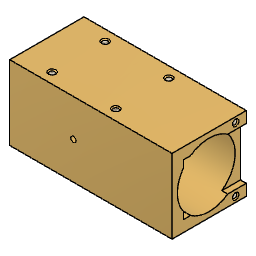
Anton_Buguev_MAM2021.01.01.000 (Autodesk Fusion 360 archive; units mm, degrees)
design "MAM2021.01.01.001"
Autodesk Fusion 360 part; units mm, degrees
sketch "Sketch1" plane through (0, 0, 0) normal (0, 1, 0) x (1, 0, 0)
  line L0 (38.25, 17.5) -> (-38.25, 17.5)
  line L1 (-38.25, 17.5) -> (-38.25, -17.5)
  line L2 (-38.25, -17.5) -> (38.25, -17.5)
  line L3 (38.25, -17.5) -> (38.25, 17.5)
  line L4 (38.25, 17.5) -> (-38.25, -17.5) construction
  line L5 (-38.25, 17.5) -> (38.25, -17.5) construction
  dimension "d1" = 76.5
  dimension "d2" = 35
  constraint horizontal L0
  constraint perpendicular L0 L1
  constraint parallel L0 L2
  constraint parallel L1 L3
  constraint coincident L4 origin
  constraint coincident L5 origin
  measures "d1" distance of L1.end L2.end
  measures "d2" distance of L0.end L1.end
extrude "Extrude1" add sketch "Sketch1" along normal blind 35
sketch "Sketch2" plane through (38.25, 0, 0) normal (1, 0, 0) x (0, 0, -1)
  line L0 (-17.5, 0) -> (17.5, 0)
  line L1 (17.5, 0) -> (17.5, 35)
  line L2 (17.5, 35) -> (-17.5, 35)
  line L3 (-17.5, 35) -> (-17.5, 0)
  circle A0 centre (0, 17.5) radius 15
  line L4 (0, 17.5) -> (17.5, 17.5) construction
  line L5 (17.5, 17.5) -> (17.5, 29.7)
  line L6 (17.5, 29.7) -> (-12, 29.7)
  line L7 (-12, 29.7) -> (-12, 5.3)
  line L8 (-12, 5.3) -> (17.5, 5.3)
  line L9 (17.5, 5.3) -> (17.5, 17.5)
  circle A1 centre (12.5, 32.5) radius 1.25 construction
  circle A2 centre (12.5, 2.5) radius 1.25 construction
  dimension "d5" = 30
  dimension "d6" = 17.5
  dimension "d7" = 17.5
  dimension "d8" = 12.2
  dimension "d9" = 29.5
  dimension "d10" = 24.4
  dimension "d11" = 2.5
  dimension "d12" = 2.5
  dimension "d13" = 5
  dimension "d14" = 2.5
  dimension "d15" = 5
  dimension "d16" = 2.5
  constraint coincident A0.centre L4.start
  constraint midpoint L1 L4.end
  constraint perpendicular L4 L5
  constraint perpendicular L5 L6
  constraint perpendicular L0 L7
  constraint coincident L1 L8.end
  constraint perpendicular L1 L8
  measures "d5" diameter of A0
  measures "d6" distance of L3 A0.centre
  measures "d7" distance of L0 A0.centre
  measures "d8" distance of L4.end L5.end
  measures "d9" distance of L5.end L6.end
  measures "d10" distance of L6.end L7.end
  measures "d11" diameter of A1
  measures "d12" distance of L2 A1.centre
  measures "d13" distance of L1 A1.centre
  measures "d14" diameter of A2
  measures "d15" distance of L1 A2.centre
  measures "d16" distance of L0 A2.centre
extrude "Extrude2" cut sketch "Sketch2" against normal blind 25.5 contours A0 L6 L7 L8 | A0 L8 | A0 L6 | A0 L7
extrude "Extrude3" cut sketch "Sketch2" against normal blind 2.75 contours L1 A0 L5 L6 L8 L9 | A0 L7 L8 | A0 L6 L7
sketch "Sketch3" plane through (-38.25, 0, 0) normal (-1, 0, 0) x (0, 0, 1)
  line L0 (-17.5, 0) -> (17.5, 0)
  line L1 (17.5, 0) -> (17.5, 35)
  line L2 (17.5, 35) -> (-17.5, 35)
  line L3 (-17.5, 35) -> (-17.5, 0)
  circle A0 centre (0, 17.5) radius 15
  line L4 (13.4987, 4.0013) -> (13.4987, 30.9987) construction
  line L5 (13.4987, 30.9987) -> (-13.4987, 30.9987) construction
  line L6 (-13.4987, 30.9987) -> (-13.4987, 4.0013) construction
  line L7 (-13.4987, 4.0013) -> (13.4987, 4.0013) construction
  circle A1 centre (-13.4987, 30.9987) radius 1.5
  circle A2 centre (13.4987, 30.9987) radius 1.5
  circle A3 centre (13.4987, 4.0013) radius 1.5
  circle A4 centre (-13.4987, 4.0013) radius 1.5
  point P0 (0, 17.5)
  dimension "d21" = 30
  dimension "d22" = 17.5
  dimension "d23" = 17.5
  dimension "d24" = 19.09
  dimension "d25" = 3
  dimension "d26" = 3
  dimension "d27" = 3
  dimension "d28" = 3
  constraint coincident P0 A0.centre
  constraint horizontal L5
  constraint coincident L5.end L6.start
  constraint coincident L4.end L5.start
  constraint coincident L4.start L7.end
  constraint coincident L6.end L7.start
  measures "d21" diameter of A0
  measures "d22" distance of L2 P0
  measures "d23" distance of L1 P0
  measures "d24" distance of L4.start P0
  measures "d25" diameter of A1
  measures "d26" diameter of A2
  measures "d27" diameter of A3
  measures "d28" diameter of A4
extrude "Extrude4" cut sketch "Sketch3" against normal blind 10 contours A0
sketch "Sketch4" plane through (-28.25, 0, 0) normal (-1, 0, 0) x (0, 0, 1)
  circle A0 centre (0, 17.5) radius 15
  circle A1 centre (0, 17.5) radius 12.5
  dimension "d31" = 25
  constraint concentric A0 A1
  measures "d31" diameter of A1
extrude "Extrude5" cut sketch "Sketch4" against normal blind 41 contours A1
sketch "Sketch5" plane through (0, 0, 17.5) normal (0, 0, 1) x (1, 0, 0)
  line L0 (-38.25, 0) -> (38.25, 0)
  line L1 (38.25, 0) -> (38.25, 35)
  line L2 (38.25, 35) -> (-38.25, 35)
  line L3 (-38.25, 35) -> (-38.25, 0)
  line L4 (-38.25, 17.5) -> (-8.25, 17.5) construction
  line L5 (-8.25, 17.5) -> (11.75, 17.5) construction
  circle A0 centre (-8.25, 17.5) radius 1.25
  circle A1 centre (11.75, 17.5) radius 2.5
  dimension "d34" = 30
  dimension "d35" = 20
  dimension "d36" = 2.5
  dimension "d37" = 5
  constraint midpoint L3 L4.start
  constraint perpendicular L3 L4
  constraint perpendicular L3 L5
  constraint coincident L4.end L5.start
  constraint coincident L5.end A1.centre
  measures "d34" distance of L4.start L4.end
  measures "d35" distance of L4.end L5.end
  measures "d36" diameter of A0
  measures "d37" diameter of A1
extrude "Extrude6" cut sketch "Sketch5" against normal blind 35 contours A0
extrude "Extrude7" cut sketch "Sketch5" along normal blind -20 and the other way blind 35 contours A1
sketch "Sketch6" plane through (0, 35, 0) normal (0, 1, 0) x (-1, 0, 0)
  line L0 (-38.25, 17.5) -> (-38.25, -17.5)
  line L1 (-38.25, -17.5) -> (38.25, -17.5)
  line L2 (38.25, -17.5) -> (38.25, 17.5)
  line L3 (38.25, 17.5) -> (-38.25, 17.5)
  circle A0 centre (23.25, -12.5) radius 1.5
  circle A1 centre (-6.75, -12.5) radius 1.5
  circle A2 centre (23.25, 12.5) radius 1.5
  circle A3 centre (-6.75, 12.5) radius 1.5
  dimension "d44" = 3
  dimension "d45" = 15
  dimension "d46" = 5
  dimension "d49" = -30
  dimension "d50" = 25
  measures "d44" diameter of A0
  measures "d45" distance of L2 A0.centre
  measures "d46" distance of L1 A0.centre
sketch "Sketch7" plane through (0, 0, 0) normal (0, -1, 0) x (1, 0, 0)
  line L0 (38.25, -17.5) -> (38.25, 17.5)
  line L1 (38.25, 17.5) -> (-38.25, 17.5)
  line L2 (-38.25, 17.5) -> (-38.25, -17.5)
  line L3 (-38.25, -17.5) -> (38.25, -17.5)
  circle A0 centre (-23.25, 12.5) radius 1.5
  circle A1 centre (6.75, 12.5) radius 1.5
  circle A2 centre (-23.25, -12.5) radius 1.5
  circle A3 centre (6.75, -12.5) radius 1.5
  dimension "d51" = 3
  dimension "d52" = 5
  dimension "d53" = 15
  dimension "d56" = 30
  dimension "d57" = -25
  measures "d51" diameter of A0
  measures "d52" distance of L1 A0.centre
  measures "d53" distance of L2 A0.centre
hole "Hole1" at (-38.25, 30.9987, 13.4987) at (-38.25, 30.9987, -13.4987) at (-38.25, 4.0013, -13.4987) at (-38.25, 4.0013, 13.4987) direction (1, 0, 0) diameter 2.529 depth 7 tip angle 118 countersink diameter 3.5 countersink angle 90
thread "Thread1" "ISO Metric profile 3.0 M3x0.5 6H" thread offset 0 thread depth 5
hole "Hole2" at (-23.25, 35, 12.5) at (6.75, 35, 12.5) at (6.75, 35, -12.5) at (-23.25, 35, -12.5) direction (0, -1, 0) diameter 2.529 depth 7 tip angle 118 countersink diameter 3.5 countersink angle 90
thread "Thread2" "ISO Metric profile 3.0 M3x0.5 6H" thread offset 0 thread depth 5
hole "Hole3" at (-23.25, 0, 12.5) at (-23.25, 0, -12.5) at (6.75, 0, -12.5) at (6.75, 0, 12.5) direction (0, 1, 0) diameter 2.529 depth 7 tip angle 118 countersink diameter 3.5 countersink angle 90
thread "Thread3" "ISO Metric profile 3.0 M3x0.5 6H" thread offset 0 thread depth 5
hole "Hole4" at (38.25, 32.5, -12.5) at (38.25, 2.5, -12.5) direction (-1, 0, 0) diameter 2.076 depth 5 tip angle 118 countersink diameter 3.05 countersink angle 90
thread "Thread4" "ISO Metric profile 2.5 M2.5x0.45 6H" thread offset 0 thread depth 4
equation "d24 = ( 38.18 / 2 ) * 1 mm"

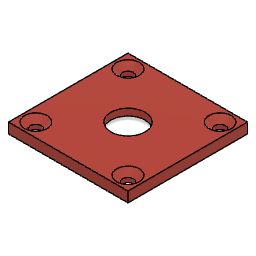
design "MAM2021.01.01.002"
Autodesk Fusion 360 part; units mm, degrees
sketch "Sketch1" plane through (0, 0, 0) normal (0, 1, 0) x (1, 0, 0)
  line L0 (17.5, -17.5) -> (-17.5, -17.5)
  line L1 (-17.5, -17.5) -> (-17.5, 17.5)
  line L2 (-17.5, 17.5) -> (17.5, 17.5)
  line L3 (17.5, 17.5) -> (17.5, -17.5)
  line L4 (17.5, -17.5) -> (-17.5, 17.5) construction
  line L5 (-17.5, -17.5) -> (17.5, 17.5) construction
  circle A0 centre (0, 0) radius 5
  dimension "d1" = 35
  dimension "d2" = 35
  dimension "d3" = 10
  constraint horizontal L0
  constraint perpendicular L0 L1
  constraint parallel L0 L2
  constraint parallel L1 L3
  constraint coincident L4 A0.centre
  constraint coincident L5 A0.centre
  constraint coincident A0.centre origin
  measures "d1" distance of L1.end L2.end
  measures "d2" distance of L0.end L1.end
  measures "d3" diameter of A0
extrude "Extrude1" add sketch "Sketch1" along normal blind 3
sketch "Sketch2" plane through (0, 3, 0) normal (0, 1, 0) x (-1, 0, 0)
  circle A0 centre (0, 0) radius 5
  line L0 (-17.5, -17.5) -> (17.5, -17.5)
  line L1 (17.5, -17.5) -> (17.5, 17.5)
  line L2 (17.5, 17.5) -> (-17.5, 17.5)
  line L3 (-17.5, 17.5) -> (-17.5, -17.5)
  line L4 (-13.4987, -13.4987) -> (13.4987, -13.4987) construction
  line L5 (13.4987, -13.4987) -> (13.4987, 13.4987) construction
  line L6 (13.4987, 13.4987) -> (-13.4987, 13.4987) construction
  line L7 (-13.4987, 13.4987) -> (-13.4987, -13.4987) construction
  circle A1 centre (0, 0) radius 10
  dimension "d6" = 19.09
  dimension "d7" = 20
  constraint coincident A0.centre A1.centre
  constraint horizontal L4
  constraint concentric A0 A1
  measures "d6" distance of L4.start A0.centre
  measures "d7" diameter of A1
hole "Hole1" at (13.4987, 3, -13.4987) at (-13.4987, 3, -13.4987) at (-13.4987, 3, 13.4987) at (13.4987, 3, 13.4987) direction (0, -1, 0) diameter 3.2 end through all countersink diameter 6.6 countersink angle 90
extrude "Extrude2" cut sketch "Sketch2" along normal blind -3 and the other way blind 2 contours A1
equation "d6 = ( 38.18 / 2 ) * 1 mm"

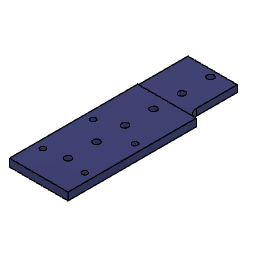
design "MAM2021.01.01.004"
Autodesk Fusion 360 part; units mm, degrees
sketch "Sketch1" plane through (0, 0, 0) normal (0, 1, 0) x (1, 0, 0)
  line L0 (0, 0) -> (17.5, 0) construction
  line L1 (17.5, -53.25) -> (17.5, 53.25)
  line L2 (17.5, 53.25) -> (-17.5, 53.25)
  line L3 (-17.5, 53.25) -> (-17.5, -23.25)
  line L4 (-17.5, -23.25) -> (-17.5, -28.75) construction
  arc A0 (-12, -28.75) -> (-17.5, -23.25) centre (-17.5, -28.75) ccw
  line L5 (-12, -28.75) -> (-12, -53.25)
  line L6 (-12, -53.25) -> (17.5, -53.25)
  line L7 (-17.5, -23.25) -> (17.5, -23.25)
  dimension "d1" = 17.5
  dimension "d2" = 106.5
  dimension "d3" = 35
  dimension "d4" = 76.5
  dimension "d5" = 5.5
  dimension "d6" = 24.5
  constraint coincident L0.start origin
  constraint horizontal L0
  constraint vertical L1
  constraint midpoint L0.end L1
  constraint perpendicular L1 L2
  constraint perpendicular L2 L3
  constraint perpendicular L2 L4
  constraint coincident L4.end A0.centre
  constraint vertical L5
  constraint perpendicular L5 L6
  constraint coincident L1 L7.end
  constraint tangent A0 L7
  measures "d1" distance of L0.start L0.end
  measures "d2" distance of L1.start L1.end
  measures "d3" distance of L1.end L2.end
  measures "d4" distance of L2.end L3.end
  measures "d5" distance of L3.end L4.end
  measures "d6" distance of A0.start L5.end
extrude "Extrude1" add sketch "Sketch1" along normal blind 4 contours L1 A0 L5 L6 L7
extrude "Extrude2" add sketch "Sketch1" along normal blind 4.5 contours L1 L2 L3 L7
sketch "Sketch2" plane through (0, 0, 0) normal (0, -1, 0) x (1, 0, 0)
  line L0 (-12, 53.25) -> (-12, 28.75)
  arc A0 (-17.5, 23.25) -> (-12, 28.75) centre (-17.5, 28.75) ccw
  line L1 (-17.5, 23.25) -> (-17.5, -53.25)
  line L2 (-17.5, -53.25) -> (17.5, -53.25)
  line L3 (17.5, -53.25) -> (17.5, 53.25)
  line L4 (17.5, 53.25) -> (-12, 53.25)
  circle A1 centre (0, 49.25) radius 2
  circle A2 centre (0, 32.25) radius 2
  circle A3 centre (0, 15.25) radius 2
  circle A4 centre (0, -1.75) radius 2
  circle A5 centre (0, -18.75) radius 2
  circle A6 centre (0, -35.75) radius 2
  circle A7 centre (12.5, -38.25) radius 1.6
  circle A8 centre (-12.5, -38.25) radius 1.6
  circle A9 centre (12.5, -8.25) radius 1.6
  circle A10 centre (-12.5, -8.25) radius 1.6
  dimension "d11" = 4
  dimension "d12" = 17.5
  dimension "d13" = 4
  dimension "d16" = 0
  dimension "d17" = -17
  dimension "d18" = 3.2
  dimension "d19" = 15
  dimension "d20" = 5
  dimension "d23" = -25
  dimension "d24" = 30
  measures "d11" diameter of A1
  measures "d12" distance of L3 A1.centre
  measures "d13" distance of L4 A1.centre
  measures "d18" diameter of A7
  measures "d19" distance of L2 A7.centre
  measures "d20" distance of L3 A7.centre
hole "Hole1" at (0, 0, 49.25) at (0, 0, 32.25) at (0, 0, 15.25) at (0, 0, -1.75) at (0, 0, -18.75) at (0, 0, -35.75) direction (0, 1, 0) diameter 4 end through all countersink diameter 5 countersink angle 90
hole "Hole2" at (12.5, 0, -8.25) at (12.5, 0, -38.25) at (-12.5, 0, -38.25) at (-12.5, 0, -8.25) direction (0, 1, 0) diameter 3.2 end through all countersink diameter 6.6 countersink angle 90
move_body "Move1" bodies 1 to x (-1, 0, 0) y (0, 1, 0) z (0, 0, -1) at (0, 0, -3.5)

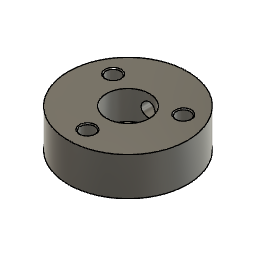
design "MAM2021.01.01.006"
Autodesk Fusion 360 part; units mm, degrees
sketch "Sketch1" plane through (0, 0, 0) normal (0, 1, 0) x (1, 0, 0)
  circle A0 centre (0, 0) radius 12.5
  circle A1 centre (0, 0) radius 4
  dimension "d1" = 25
  dimension "d2" = 8
  constraint coincident A0.centre A1.centre
  constraint concentric A0 A1
  measures "d1" diameter of A0
  measures "d2" diameter of A1
extrude "Extrude1" add sketch "Sketch1" along normal blind 8
sketch "Sketch2" plane through (0, 8, 0) normal (0, 1, 0) x (-1, 0, 0)
  circle A0 centre (0, 0) radius 4
  circle A1 centre (0, 0) radius 12.5
  circle A2 centre (0, 0) radius 8.5 construction
  line L0 (0, 0) -> (0, 8.5) construction
  circle A3 centre (0, 8.5) radius 1.5 construction
  circle A4 centre (-7.3612, -4.25) radius 1.5 construction
  circle A5 centre (7.3612, -4.25) radius 1.5 construction
  circle A6 centre (0, 0) radius 4.5 construction
  dimension "d5" = 17
  dimension "d6" = 3
  dimension "d8" = 360
  dimension "d9" = 9
  constraint coincident A0.centre A1.centre
  constraint coincident A2 L0.end
  constraint vertical L0
  constraint coincident L0.end A3.centre
  measures "d5" diameter of A2
  measures "d6" diameter of A3
  measures "d9" diameter of A6
hole "Hole1" at (0, 8, 8.5) at (-7.3612, 8, -4.25) at (7.3612, 8, -4.25) direction (0, -1, 0) diameter 3 end through all countersink diameter 3.4 countersink angle 90
hole "Hole2" at (0, 8, 0) direction (0, -1, 0) diameter 9 depth 6 tip angle 180
ref_plane "WorkPlane1" through (0, 0, -12.5) normal (0, 0, 1) x (1, 0, 0)
sketch "Sketch3" plane through (0, 0, -12.5) normal (0, 0, 1) x (1, 0, 0)
  circle A0 centre (0, 5) radius 1.5
  line L0 (0, 0) -> (0, 5) construction
  dimension "d19" = 3
  dimension "d20" = 5
  constraint coincident L0.start origin
  constraint coincident A0.centre L0.end
  constraint vertical L0
  measures "d19" diameter of A0
  measures "d20" distance of L0.start A0.centre
extrude "Extrude2" cut sketch "Sketch3" along normal blind 9
chamfer "Chamfer1" distance 0.2 angle 45 2 edges at (-1.5, 5, -12.4097) (1.5, 5, -12.4097) measured on face at (12.4379, 2.6667, 1.2446) measured on face at (12.4379, 2.6667, 1.2446)

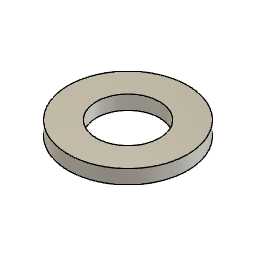
design "MAM2021.01.03.001"
Autodesk Fusion 360 part; units mm, degrees
sketch "Sketch1" plane through (0, 0, 0) normal (0, 1, 0) x (1, 0, 0)
  circle A0 centre (0, 0) radius 8.5
  circle A1 centre (0, 0) radius 4.5
  dimension "d1" = 17
  dimension "d2" = 9
  constraint coincident A0.centre A1.centre
  constraint concentric A0 A1
  measures "d1" diameter of A0
  measures "d2" diameter of A1
extrude "Extrude1" add sketch "Sketch1" along normal blind 2

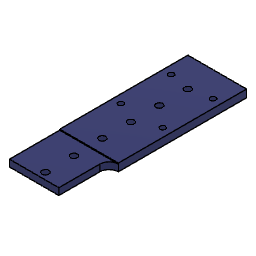
design "MAM2021.01.01.003"
Autodesk Fusion 360 part; units mm, degrees
sketch "Sketch1" plane through (0, 0, 0) normal (0, 1, 0) x (1, 0, 0)
  line L0 (0, 0) -> (-17.5, 0) construction
  line L1 (-17.5, -53.25) -> (-17.5, 53.25)
  line L2 (-17.5, 53.25) -> (17.5, 53.25)
  line L3 (17.5, 53.25) -> (17.5, -23.25)
  line L4 (17.5, -23.25) -> (17.5, -28.75) construction
  arc A0 (17.5, -23.25) -> (12, -28.75) centre (17.5, -28.75) ccw
  line L5 (17.5, -28.75) -> (17.5, -23.25) construction
  line L6 (17.5, -28.75) -> (12, -28.75) construction
  line L7 (12, -28.75) -> (12, -53.25)
  line L8 (12, -53.25) -> (-17.5, -53.25)
  line L9 (17.5, -23.25) -> (-17.5, -23.25)
  dimension "d1" = 17.5
  dimension "d2" = 106.5
  dimension "d3" = 35
  dimension "d4" = 76.5
  dimension "d5" = 5.5
  dimension "d6" = 90
  dimension "d7" = 24.5
  constraint coincident L0.start origin
  constraint horizontal L0
  constraint vertical L1
  constraint midpoint L0.end L1
  constraint perpendicular L1 L2
  constraint perpendicular L2 L3
  constraint perpendicular L2 L4
  constraint coincident L4.end A0.centre
  constraint perpendicular L6 L7
  constraint coincident L1 L9.end
  constraint tangent A0 L9
  measures "d1" distance of L0.start L0.end
  measures "d2" distance of L1.start L1.end
  measures "d3" distance of L1.end L2.end
  measures "d4" distance of L2.end L3.end
  measures "d5" distance of L3.end L4.end
  measures "d6" angle of L5 L6
  measures "d7" distance of A0.end L7.end
extrude "Extrude1" add sketch "Sketch1" along normal blind 4 contours L1 A0 L7 L8 L9
extrude "Extrude2" add sketch "Sketch1" along normal blind 4.5 contours L1 L2 L3 L9
sketch "Sketch2" plane through (0, 0, 0) normal (0, -1, 0) x (1, 0, 0)
  arc A0 (12, 28.75) -> (17.5, 23.25) centre (17.5, 28.75) ccw
  line L0 (12, 28.75) -> (12, 53.25)
  line L1 (12, 53.25) -> (-17.5, 53.25)
  line L2 (-17.5, 53.25) -> (-17.5, -53.25)
  line L3 (-17.5, -53.25) -> (17.5, -53.25)
  line L4 (17.5, -53.25) -> (17.5, 23.25)
  circle A1 centre (0, 49.25) radius 2
  circle A2 centre (0, 32.25) radius 2
  circle A3 centre (0, 15.25) radius 2
  circle A4 centre (0, -1.75) radius 2
  circle A5 centre (0, -18.75) radius 2
  circle A6 centre (0, -35.75) radius 2
  circle A7 centre (-12.5, -38.25) radius 1.6
  circle A8 centre (12.5, -38.25) radius 1.6
  circle A9 centre (-12.5, -8.25) radius 1.6
  circle A10 centre (12.5, -8.25) radius 1.6
  dimension "d12" = 4
  dimension "d13" = 17.5
  dimension "d14" = 4
  dimension "d17" = 0
  dimension "d18" = -17
  dimension "d19" = 3.2
  dimension "d20" = 15
  dimension "d21" = 5
  dimension "d24" = 25
  dimension "d25" = 30
  measures "d12" diameter of A1
  measures "d13" distance of L2 A1.centre
  measures "d14" distance of L1 A1.centre
  measures "d19" diameter of A7
  measures "d20" distance of L3 A7.centre
  measures "d21" distance of L2 A7.centre
hole "Hole1" at (0, 0, 49.25) at (0, 0, 32.25) at (0, 0, 15.25) at (0, 0, -1.75) at (0, 0, -18.75) at (0, 0, -35.75) direction (0, 1, 0) diameter 4 end through all countersink diameter 4.4 countersink angle 90
hole "Hole2" at (12.5, 0, -8.25) at (12.5, 0, -38.25) at (-12.5, 0, -38.25) at (-12.5, 0, -8.25) direction (0, 1, 0) diameter 3.2 end through all countersink diameter 6.6 countersink angle 90
